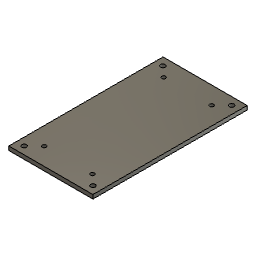
Cube Base (Autodesk Fusion 360 design; units mm, degrees)
Autodesk Fusion 360 part; units mm, degrees
note: some values were not read from the file. Set by a fixed rule: which sketch regions a step uses.
sketch "Sketch1" plane through (0, 0, 0) normal (0, 1, 0) x (1, 0, 0)
  circle A0 centre (0.5, 99.5) radius 1.6662
  circle A1 centre (7.805, 92.54) radius 1.375
  circle A2 centre (42.195, 92.54) radius 1.375
  circle A3 centre (49.5, 99.5) radius 1.6662
  circle A4 centre (7.805, 7.46) radius 1.375
  circle A5 centre (0.5, 0.5) radius 1.6662
  circle A6 centre (42.195, 7.46) radius 1.375
  circle A7 centre (49.5, 0.5) radius 1.6662
  line L0 (-5, -5) -> (55, -5)
  line L1 (55, -5) -> (55, 105)
  line L2 (55, 105) -> (-5, 105)
  line L3 (-5, 105) -> (-5, -5)
  dimension "d5" = 3.3325
  dimension "d8" = 2.75
  measures "d5" diameter of A0
  measures "d8" diameter of A1
extrude "Extrude1" add sketch "Sketch1" along normal blind 2.794
